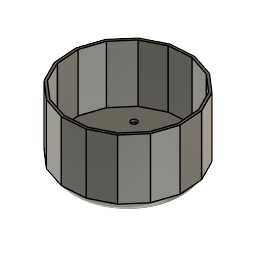
Untitled1 (Autodesk Fusion 360 design; units mm, degrees)
part number: 2026-01-26-19-48-44-269
Autodesk Fusion 360 part; units mm, degrees
sketch "Sketch1" plane through (0, 0, 0) normal (0, 0, 1) x (1, 0, 0)
  line L0 (43.4762, -24.6945) -> (49.617, -6.1771)
  line L1 (49.617, -6.1771) -> (48.204, 13.2807)
  line L2 (48.204, 13.2807) -> (39.4524, 30.7166)
  line L3 (39.4524, 30.7166) -> (24.6945, 43.4762)
  line L4 (24.6945, 43.4762) -> (6.1771, 49.617)
  line L5 (6.1771, 49.617) -> (-13.2807, 48.204)
  line L6 (-13.2807, 48.204) -> (-30.7166, 39.4524)
  line L7 (-30.7166, 39.4524) -> (-43.4762, 24.6945)
  line L8 (-43.4762, 24.6945) -> (-49.617, 6.1771)
  line L9 (-49.617, 6.1771) -> (-48.204, -13.2807)
  line L10 (-48.204, -13.2807) -> (-39.4524, -30.7166)
  line L11 (-39.4524, -30.7166) -> (-24.6945, -43.4762)
  line L12 (-24.6945, -43.4762) -> (-6.1771, -49.617)
  line L13 (-6.1771, -49.617) -> (13.2807, -48.204)
  line L14 (13.2807, -48.204) -> (30.7166, -39.4524)
  line L15 (30.7166, -39.4524) -> (43.4762, -24.6945)
extrude "Extrude1" add sketch "Sketch1" along normal blind 50 makes body 1
sketch "Sketch2" plane through (0, 0, 50) normal (0, 0, 1) x (-1, 0, 0)
  line L0 (-30.7166, 39.4524) -> (-43.4762, 24.6945)
  line L1 (-43.4762, 24.6945) -> (-49.617, 6.1771)
  line L2 (-49.617, 6.1771) -> (-48.204, -13.2807)
  line L3 (-48.204, -13.2807) -> (-39.4524, -30.7166)
  line L4 (-39.4524, -30.7166) -> (-24.6945, -43.4762)
  line L5 (-24.6945, -43.4762) -> (-6.1771, -49.617)
  line L6 (-6.1771, -49.617) -> (13.2807, -48.204)
  line L7 (13.2807, -48.204) -> (30.7166, -39.4524)
  line L8 (30.7166, -39.4524) -> (43.4762, -24.6945)
  line L9 (43.4762, -24.6945) -> (49.617, -6.1771)
  line L10 (49.617, -6.1771) -> (48.204, 13.2807)
  line L11 (48.204, 13.2807) -> (39.4524, 30.7166)
  line L12 (39.4524, 30.7166) -> (24.6945, 43.4762)
  line L13 (24.6945, 43.4762) -> (6.1771, 49.617)
  line L14 (6.1771, 49.617) -> (-13.2807, 48.204)
  line L15 (-13.2807, 48.204) -> (-30.7166, 39.4524)
  circle A0 centre (-135, 0) radius 47.5
  dimension "d4" = 95
  measures "d4" diameter of A0
extrude "Extrude2" add sketch "Sketch2" along normal blind 10 separate body contours A0 makes body 2
fillet "Fillet1" radius 10 1 edges at (179.2855, 17.1767, 50) on bodies 2
move_body "Move1" bodies 2 to x (1, 0, 0) y (0, 1, 0) z (0, 0, 1) at (-135, 0, -60)
shell "Shell1" thickness 2 removed faces 1 at (10.2389, -13.1508, 50) on bodies 1
sketch "Sketch3" plane through (0, 0, 2) normal (0, 0, 1) x (-1, 0, 0)
  line L0 (-29.4639, 37.8434) -> (-41.7031, 23.6874)
  line L1 (-41.7031, 23.6874) -> (-47.5934, 5.9252)
  line L2 (-47.5934, 5.9252) -> (-46.238, -12.7391)
  line L3 (-46.238, -12.7391) -> (-37.8434, -29.4639)
  line L4 (-37.8434, -29.4639) -> (-23.6874, -41.7031)
  line L5 (-23.6874, -41.7031) -> (-5.9252, -47.5934)
  line L6 (-5.9252, -47.5934) -> (12.7391, -46.238)
  line L7 (12.7391, -46.238) -> (29.4639, -37.8434)
  line L8 (29.4639, -37.8434) -> (41.7031, -23.6874)
  line L9 (41.7031, -23.6874) -> (47.5934, -5.9252)
  line L10 (47.5934, -5.9252) -> (46.238, 12.7391)
  line L11 (46.238, 12.7391) -> (37.8434, 29.4639)
  line L12 (37.8434, 29.4639) -> (23.6874, 41.7031)
  line L13 (23.6874, 41.7031) -> (5.9252, 47.5934)
  line L14 (5.9252, 47.5934) -> (-12.7391, 46.238)
  line L15 (-12.7391, 46.238) -> (-29.4639, 37.8434)
  circle A0 centre (20, -25) radius 2.5
  dimension "d10" = 5
  measures "d10" diameter of A0
extrude "Extrude3" cut sketch "Sketch3" against normal blind 110 contours A0 bodies 1 2
